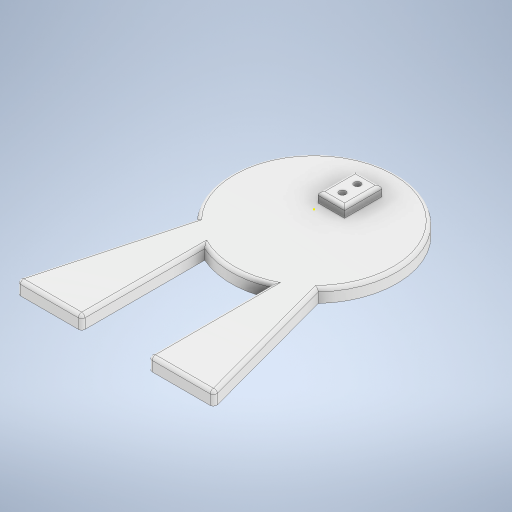
# Autodesk Inventor part: Base inferior(suporte)
Saved by Autodesk Inventor 2023 (Build 270158000, 158)
## iProperties
Created: 2023-03-10
Part Number: Base inferior(suporte)
Material: ABS Plastic
Document SubType Name: Modeling
Designer: Antonio Ribeiro
Density: 1.06 g/cm^3
Appearance: Smooth - White
Author: Antonio Ribeiro
## iProperties of the stored document Base inferior(suporte)_3DPrint.ipt
Created: 2023-03-28
Part Number: Base inferior(suporte)_3DPrint
Material: Generic
Document SubType Name: Modeling
Designer: Inteli
Density: 1 g/cm^3
Appearance: Default
Author: Inteli
Autodesk Inventor part; units mm, degrees
ref_plane "YZ Plane" through (0, 0, 0) normal (1, 0, 0) x (0, 1, 0)
ref_plane "XZ Plane" through (0, 0, 0) normal (0, 1, 0) x (-1, 0, 0)
ref_plane "XY Plane" through (0, 0, 0) normal (0, 0, 1) x (1, 0, 0)
sketch "Esboço1" plane through (0, 0, 0) normal (0, 1, 0) x (-1, 0, 0)
  line L0 (-20.2851, 120) -> (-59.8779, 120)
  line L1 (-36.6213, 34.0423) -> (-59.8779, 120)
  line L2 (20.2851, 120) -> (59.878, 120)
  line L3 (59.878, 120) -> (36.6213, 34.0423)
  line L4 (20.2851, 45.7003) -> (20.2851, 120)
  line L5 (-20.2851, 45.7003) -> (-20.2851, 120)
  arc A0 (20.2851, 45.7003) -> (-20.2851, 45.7003) centre (0, 0) ccw
  arc A1 (-36.6213, 34.0423) -> (36.6213, 34.0423) centre (0, 0) ccw
  constraints: 12 end point, 4 point on circle, 2 centre point, 2 perpendicular, 1 coincident, 1 point on line
extrude "Extrusão1" add sketch "Esboço1" along normal blind 8
sketch "Sketch9" plane through (0, 8, 0) normal (0, 1, 0) x (1, 0, 0)
  arc A0 (36.6213, -34.0423) -> (-36.6213, -34.0423) centre (0, 0) ccw projected
  line L0 (-8, 15) -> (-8, 12)
  line L1 (8, 12) -> (8, 33)
  line L2 (8, 33) -> (-8, 33)
  line L3 (-8, 33) -> (-8, 15)
  line L4 (-8, 12) -> (-8, 10.5)
  line L5 (-8, 10.5) -> (8, 10.5)
  line L6 (8, 10.5) -> (8, 12)
  point P0 (5, 30)
  point P1 (5, 15)
  point P2 (-5, 15)
  dimension "d34" = 3
  dimension "d36" = 21
  dimension "d37" = 16
  dimension "d49" = 1.5
  constraints: 14 end point, 2 perpendicular, 1 vertical
  measures "d34" distance of L0.start L0.end
  measures "d36" distance of L1.start L1.end
  measures "d37" distance of L1.end L2.end
  measures "d49" distance of L0.end L4.end
extrude "Extrusion5" add sketch "Sketch9" along normal blind 6
sketch "Sketch10" plane through (0, 14, 0) normal (0, 1, 0) x (1, 0, 0)
  line L0 (-8, 33) -> (8, 33) projected
  line L1 (-8, 12) -> (8, 12) projected
  circle A0 centre (0, 17.25) radius 3.5
  circle A1 centre (0, 26.25) radius 3.5
  point P0 (0, 0)
  dimension "d57" = 7
  dimension "d58" = 7
  constraints: 2 centre point
  measures "d57" diameter of A0
  measures "d58" diameter of A1
extrude "Extrusion6" [suppressed]
fillet "Fillet2" radius 2 4 edges at (0, 14, -10.5) (8, 14, -21.75) (-8, 14, -21.75) (0, 14, -33)
sketch "Sketch12" plane through (0, 14, 0) normal (0, 1, 0) x (1, 0, 0)
  point P0 (0, 0)
sketch "Sketch13" plane through (0, 0, 0) normal (0, -1, 0) x (1, 0, 0)
  line L0 (8, -33) -> (8, -10.5) projected
  line L1 (8, -10.5) -> (-8, -10.5) projected
  line L2 (8, -10.5) -> (-8, -10.5)
  line L3 (-8, -10.5) -> (-8, -33) projected
  line L4 (-8, -10.5) -> (-8, -33)
  line L5 (-8, -33) -> (8, -33) projected
  line L6 (-8, -33) -> (8, -33)
  line L7 (8, -33) -> (8, -10.5)
  point P0 (0, 0)
  constraints: 8 end point, 3 collinear, 1 perpendicular
extrude "Extrusion7" cut sketch "Sketch13" against normal blind 3
fillet "Fillet3" radius 6 4 edges at (-8, 0, -21.75) (0, 0, -33) (8, 0, -21.75) (0, 0, -10.5)
sketch "Sketch14" plane through (0, 3, 0) normal (0, -1, 0) x (1, 0, 0)
  circle A0 centre (0, -17.25) radius 2 projected
  circle A1 centre (0, -17.25) radius 2
  circle A2 centre (0, -26.25) radius 2 projected
  circle A3 centre (0, -26.25) radius 2
  point P0 (0, 0)
  constraints: 2 centre point, 2 coincident
extrude "Extrusion8" cut sketch "Sketch14" against normal through all
fillet "Fillet4" radius 1 2 edges at (-2, 3, -17.25) (-2, 3, -26.25)
fillet "Fillet5" radius 2 8 edges at (0, 8, -50) (48.2496, 8, 77.0212) (0, 8, 50) (20.2851, 8, 82.8501) (40.0815, 8, 120) (-48.2497, 8, 77.0212) (-20.2851, 8, 82.8501) (-40.0816, 8, 120)
fillet "Fillet6" radius 2 8 edges at (-59.1127, 7.4142, 119.4142) (-59.878, 3, 120) (-20.8709, 7.4142, 119.4142) (-20.2851, 3, 120) (20.2851, 3, 120) (20.8709, 7.4142, 119.4142) (59.1126, 7.4142, 119.4142) (59.8779, 3, 120)
